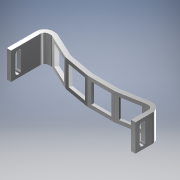
# Autodesk Inventor part: key_holder_metal
Saved by Autodesk Inventor 2018 (Build 220112000, 112)
## iProperties
Created: 2018-04-04
Part Number: key_holder_metal
Material: アルミニウム 6061
Document SubType Name: Sheet Metal
Designer: NaMACHAN
Density: 2.7 g/cm^3
Sheet Metal Rule: Default_mm
Appearance: アルミニウム - フラット
Mass: 6.46479 g
Surface Area: 40.6835 cm^2
Volume: 2.39437 cm^3
Author: NaMACHAN
Autodesk Inventor part; units mm, degrees
ref_plane "YZ Plane" through (0, 0, 0) normal (1, 0, 0) x (0, 1, 0)
ref_plane "XZ Plane" through (0, 0, 0) normal (0, 1, 0) x (-1, 0, 0)
ref_plane "XY Plane" through (0, 0, 0) normal (0, 0, 1) x (1, 0, 0)
sketch "スケッチ2" plane through (0, 0, 0) normal (0, 1, 0) x (-1, 0, 0)
  line L0 (-9.5, -9.5) -> (9.5, -9.5)
  line L1 (9.5, -9.5) -> (9.5, 9.5)
  line L2 (9.5, 9.5) -> (-9.5, 9.5)
  line L3 (-9.5, 9.5) -> (-9.5, -9.5)
  line L4 (-9.5, -9.5) -> (9.5, 9.5) construction
  line L5 (9.5, -9.5) -> (-9.5, 9.5) construction
  point P0 (0, 0)
  dimension "d4" = 19
  dimension "d5" = 19
  measures "d4" distance of L2.end L1.end
  measures "d5" distance of L1.end L0.end
extrude "プレート1" add sketch "スケッチ2" along normal blind 3
sketch "スケッチ3" plane through (8.9791, 2.9544, -9.5) normal (0.1736482, -0.9848078, 0) x (0.9848078, 0.1736482, 0)
  line L0 (0, 19) -> (0, 0)
  line L1 (0, 0) -> (19, 0)
  line L2 (19, 0) -> (19, 19)
  line L3 (19, 19) -> (0, 19)
  constraints: 6 end point, 1 horizontal, 1 perpendicular, 1 vertical
edge flange "フランジ1" height 19 angle 10 thickness 3 bend radius 3 thickness toward (0.1736482, -0.9848078, 0) relief straight relief width 3 relief depth 1.5 edges at (9.5, 3, 0) wall of the first edge with corners at (8.9791, 2.9544, 9.5) (8.9791, 2.9544, -9.5) (27.6904, 6.2537, -9.5) (27.6904, 6.2537, 9.5)
bend "曲げ1"
corner "コーナー1"
sketch "スケッチ4" plane through (-8.9791, 2.9544, 9.5) normal (-0.1736482, -0.9848078, 0) x (0.9848078, -0.1736482, 0)
  line L0 (0, -19) -> (0, 0)
  line L1 (0, 0) -> (-19, 0)
  line L2 (-19, 0) -> (-19, -19)
  line L3 (-19, -19) -> (0, -19)
  constraints: 6 end point, 1 horizontal, 1 perpendicular, 1 vertical
edge flange "フランジ2" height 19 angle 10 thickness 3 bend radius 3 thickness toward (-0.1736482, -0.9848078, 0) relief straight relief width 3 relief depth 1.5 edges at (-9.5, 3, 0) wall of the first edge with corners at (-8.9791, 2.9544, -9.5) (-8.9791, 2.9544, 9.5) (-27.6904, 6.2537, 9.5) (-27.6904, 6.2537, -9.5)
bend "曲げ2"
corner "コーナー2"
sketch "スケッチ5" plane through (-26.9435, 6.0182, 9.5) normal (-0.4226183, -0.9063078, 0) x (0.9063078, -0.4226183, 0)
  line L0 (0, -19) -> (0, 0)
  line L1 (0, 0) -> (-19.395, 0)
  line L2 (-19.395, 0) -> (-19.395, -19)
  line L3 (-19.395, -19) -> (0, -19)
  constraints: 6 end point, 1 horizontal, 1 perpendicular, 1 vertical
edge flange "フランジ3" height 19 angle 15 thickness 3 bend radius 3 thickness toward (-0.4226183, -0.9063078, 0) relief straight relief width 3 relief depth 1.5 edges at (-27.6904, 6.2537, 0) wall of the first edge with corners at (-26.9435, 6.0182, -9.5) (-26.9435, 6.0182, 9.5) (-44.5213, 14.2149, 9.5) (-44.5213, 14.2149, -9.5)
bend "曲げ3"
corner "コーナー3"
sketch "スケッチ11" plane through (9.496, 3.0456, 9.5) normal (-0.1736482, 0.9848078, 0) x (0.9848078, 0.1736482, 0)
  line L0 (0.9751, 17.5) -> (16.9751, 17.5)
  line L1 (16.9751, 17.5) -> (16.9751, 1.5)
  line L2 (16.9751, 1.5) -> (0.9751, 1.5)
  line L3 (0.9751, 1.5) -> (0.9751, 17.5)
  line L4 (0.9751, 17.5) -> (16.9751, 1.5) construction
  line L5 (16.9751, 17.5) -> (0.9751, 1.5) construction
  line L6 (18.4751, 0) -> (0, 0) projected
  line L7 (0, 19) -> (0, 0) projected
  point P0 (-9.8806, 9.5)
  point P1 (8.9751, 9.5)
  point P2 (8.9751, 9.5)
  point P3 (20.4467, 9.5)
  point P4 (8.9751, 9.5)
  point P5 (8.9751, 0)
  point P6 (17.9501, 0)
  point P7 (0, 9.5)
  dimension "d87" = 16
  dimension "d88" = 16
  constraints: 12 end point, 5 midpoint, 2 horizontal alignment, 2 parallel, 1 horizontal, 1 perpendicular, 1 point on line, 1 vertical alignment
  measures "d87" distance of L1.end L2.end
  measures "d88" distance of L0.end L1.end
extrude "押し出し2" cut sketch "スケッチ11" against normal blind 1.5
sketch "スケッチ12" plane through (0, 3, 0) normal (0, 1, 0) x (1, 0, 0)
  line L0 (-8, 8) -> (8, 8)
  line L1 (8, 8) -> (8, -8)
  line L2 (8, -8) -> (-8, -8)
  line L3 (-8, -8) -> (-8, 8)
  line L4 (-8, 8) -> (8, -8) construction
  line L5 (8, 8) -> (-8, -8) construction
  point P0 (0, 0)
  dimension "d91" = 16
  dimension "d92" = 16
  constraints: 12 end point, 2 midpoint, 2 parallel, 1 horizontal, 1 perpendicular
  measures "d91" distance of L1.end L2.end
  measures "d92" distance of L0.end L1.end
extrude "押し出し3" cut sketch "スケッチ12" against normal blind 1.5
sketch "スケッチ13" plane through (-9.496, 3.0456, 9.5) normal (0.1736482, 0.9848078, 0) x (0.9848078, -0.1736482, 0)
  line L0 (-0.8426, 17.5) -> (-16.8426, 17.5)
  line L1 (-16.8426, 17.5) -> (-16.8426, 1.5)
  line L2 (-16.8426, 1.5) -> (-0.8426, 1.5)
  line L3 (-0.8426, 1.5) -> (-0.8426, 17.5)
  line L4 (-0.8426, 17.5) -> (-16.8426, 1.5) construction
  line L5 (-16.8426, 17.5) -> (-0.8426, 1.5) construction
  line L6 (-17.6852, 19) -> (0, 19) projected
  line L7 (0.5209, 19) -> (0.5209, 0) projected
  point P0 (9.8806, 9.5)
  point P1 (-8.8426, 9.5)
  point P2 (-8.8426, 9.5)
  point P3 (-0.8426, 9.5)
  point P4 (-8.8426, 9.5)
  point P5 (-8.8426, 19)
  point P6 (0.5209, 9.5)
  dimension "d95" = 16
  dimension "d96" = 16
  constraints: 12 end point, 7 midpoint, 2 horizontal alignment, 2 parallel, 1 horizontal, 1 perpendicular, 1 vertical alignment
  measures "d95" distance of L2.end L1.end
  measures "d96" distance of L1.end L0.end
extrude "押し出し4" cut sketch "スケッチ13" against normal blind 1.5
sketch "スケッチ14" plane through (-27.6594, 6.3521, 9.5) normal (0.4226183, 0.9063078, 0) x (0.9063078, -0.4226183, 0)
  line L0 (-0.6374, 17.5) -> (-16.6374, 17.5)
  line L1 (-16.6374, 17.5) -> (-16.6374, 1.5)
  line L2 (-16.6374, 1.5) -> (-0.6374, 1.5)
  line L3 (-0.6374, 1.5) -> (-0.6374, 17.5)
  line L4 (-0.6374, 17.5) -> (-16.6374, 1.5) construction
  line L5 (-16.6374, 17.5) -> (-0.6374, 1.5) construction
  line L6 (-18.605, 19) -> (0, 19) projected
  line L7 (0, 0) -> (0, 19) projected
  point P0 (27.7524, 9.5)
  point P1 (-8.6374, 9.5)
  point P2 (-8.6374, 9.5)
  point P3 (-8.6374, 19)
  point P4 (-17.2749, 19)
  point P5 (-8.6374, 9.5)
  point P6 (0, 9.5)
  dimension "d99" = 16
  dimension "d100" = 16
  constraints: 12 end point, 5 midpoint, 2 parallel, 1 horizontal, 1 horizontal alignment, 1 perpendicular, 1 point on line, 1 vertical alignment
  measures "d99" distance of L2.end L1.end
  measures "d100" distance of L1.end L0.end
extrude "押し出し5" cut sketch "スケッチ14" against normal blind 1.5
sketch "スケッチ18" plane through (28.7323, 3.3449, -9.5) normal (0, 1, 0) x (1, 0, 0)
  line L0 (0, 19) -> (0, 0)
  line L1 (0, 0) -> (6.8755, 0)
  line L2 (6.8755, 0) -> (6.8755, 19)
  line L3 (6.8755, 19) -> (0, 19)
  constraints: 6 end point, 1 horizontal, 1 perpendicular, 1 vertical
edge flange "フランジ9" height 7.138 angle -10 thickness 3 bend radius 3 thickness toward (0, 1, 0) relief straight relief width 3 relief depth 1.5 edges at (27.6904, 6.2537, 0) wall of the first edge with corners at (28.7323, 3.3449, 9.5) (28.7323, 3.3449, -9.5) (35.6078, 3.3449, -9.5) (35.6078, 3.3449, 9.5)
bend "曲げ9"
corner "コーナー9"
sketch "スケッチ19" plane through (-47.057, 11.7771, 9.5) normal (0, 1, 0) x (1, 0, 0)
  line L0 (0, -19) -> (0, 0)
  line L1 (0, 0) -> (-7.3349, 0)
  line L2 (-7.3349, 0) -> (-7.3349, -19)
  line L3 (-7.3349, -19) -> (0, -19)
  constraints: 6 end point, 1 horizontal, 1 perpendicular, 1 vertical
edge flange "フランジ10" height 8 angle -25 thickness 3 bend radius 3 thickness toward (0, 1, 0) relief straight relief width 3 relief depth 1.5 edges at (-44.5213, 14.2149, 0) wall of the first edge with corners at (-47.057, 11.7771, -9.5) (-47.057, 11.7771, 9.5) (-54.3919, 11.7771, 9.5) (-54.3919, 11.7771, -9.5)
bend "曲げ10"
corner "コーナー10"
sketch "スケッチ20" plane through (32.6078, 6.3449, -9.5) normal (1, 0, 0) x (0, -1, 0)
  line L0 (0, 19) -> (0, 0)
  line L1 (0, 0) -> (18, 0)
  line L2 (18, 0) -> (18, 19)
  line L3 (18, 19) -> (0, 19)
  constraints: 6 end point, 1 horizontal, 1 perpendicular, 1 vertical
edge flange "フランジ11" height 15 angle -90 thickness 3 bend radius 3 thickness toward (1, 0, 0) relief straight relief width 3 relief depth 1.5 edges at (35.6078, 6.3449, 0) wall of the first edge with corners at (32.6078, 6.3449, 9.5) (32.6078, 6.3449, -9.5) (32.6078, -11.6551, -9.5) (32.6078, -11.6551, 9.5)
bend "曲げ11"
corner "コーナー11"
sketch "スケッチ21" plane through (-51.3919, 14.7771, 9.5) normal (-1, 0, 0) x (0, 1, 0)
  line L0 (0, -19) -> (0, 0)
  line L1 (0, 0) -> (-26.432, 0)
  line L2 (-26.432, 0) -> (-26.432, -19)
  line L3 (-26.432, -19) -> (0, -19)
  constraints: 6 end point, 1 horizontal, 1 perpendicular, 1 vertical
edge flange "フランジ12" height 23.432 angle -90 thickness 3 bend radius 3 thickness toward (-1, 0, 0) relief straight relief width 3 relief depth 1.5 edges at (-54.3919, 14.7771, 0) wall of the first edge with corners at (-51.3919, 14.7771, -9.5) (-51.3919, 14.7771, 9.5) (-51.3919, -11.6549, 9.5) (-51.3919, -11.6549, -9.5)
bend "曲げ12"
corner "コーナー12"
sketch "スケッチ22" plane through (35.6078, -11.6551, 9.5) normal (1, 0, 0) x (0, 0, -1)
  line L0 (4, 7) -> (15, 7)
  arc A0 (15, 3) -> (15, 7) centre (15, 5) ccw
  line L1 (15, 3) -> (4, 3)
  arc A1 (4, 7) -> (4, 3) centre (4, 5) ccw
  line L2 (0, 12) -> (0, 0) projected
  line L3 (19, 12) -> (19, 0) projected
  line L4 (0, 0) -> (19, 0) projected
  dimension "d194" = 2
  dimension "d195" = 4
  dimension "d196" = 4
  dimension "d197" = 5
  constraints: 4 end point, 4 point on circle, 4 tangent, 2 centre point, 1 horizontal, 1 parallel
  measures "d194" radius of A1
  measures "d195" distance from line of L2 A1.centre
  measures "d196" distance from line of L3 A0.centre
  measures "d197" distance from line of L4 A0.centre
extrude "押し出し8" cut sketch "スケッチ22" against normal blind 100
sketch "スケッチ23" plane through (9.7565, 1.5684, 9.5) normal (-0.1736482, 0.9848078, 0) x (0.9848078, 0.1736482, 0)
  line L0 (1.9751, 2.5) -> (15.9751, 2.5)
  line L1 (15.9751, 2.5) -> (15.9751, 16.5)
  line L2 (15.9751, 16.5) -> (1.9751, 16.5)
  line L3 (1.9751, 16.5) -> (1.9751, 2.5)
  line L4 (1.9751, 2.5) -> (15.9751, 16.5) construction
  line L5 (15.9751, 2.5) -> (1.9751, 16.5) construction
  line L6 (16.9751, 17.5) -> (16.9751, 1.5) projected
  line L7 (16.9751, 1.5) -> (0.9751, 1.5) projected
  point P0 (-9.8806, 9.5)
  point P1 (8.9751, 9.5)
  point P2 (8.9751, 9.5)
  point P3 (16.9751, 9.5)
  point P4 (8.9751, 9.5)
  point P5 (8.9751, 2.5)
  point P6 (8.9751, 1.5)
  dimension "d178" = 14
  dimension "d179" = 14
  constraints: 12 end point, 7 midpoint, 2 parallel, 2 vertical alignment, 1 horizontal, 1 horizontal alignment, 1 perpendicular
  measures "d178" distance of L2.end L1.end
  measures "d179" distance of L1.end L0.end
extrude "押し出し9" cut sketch "スケッチ23" against normal blind 1.5
sketch "スケッチ24" plane through (0, 1.5, 0) normal (0, 1, 0) x (1, 0, 0)
  line L0 (-7, -7) -> (7, -7)
  line L1 (7, -7) -> (7, 7)
  line L2 (7, 7) -> (-7, 7)
  line L3 (-7, 7) -> (-7, -7)
  line L4 (-7, -7) -> (7, 7) construction
  line L5 (7, -7) -> (-7, 7) construction
  point P0 (0, 0)
  dimension "d182" = 14
  dimension "d183" = 14
  constraints: 12 end point, 2 midpoint, 2 parallel, 1 horizontal, 1 perpendicular
  measures "d182" distance of L2.end L1.end
  measures "d183" distance of L1.end L0.end
extrude "押し出し10" cut sketch "スケッチ24" against normal blind 1.5
sketch "スケッチ25" plane through (-9.7565, 1.5684, 9.5) normal (0.1736482, 0.9848078, 0) x (0.9848078, -0.1736482, 0)
  line L0 (-15.8426, 2.5) -> (-1.8426, 2.5)
  line L1 (-1.8426, 2.5) -> (-1.8426, 16.5)
  line L2 (-1.8426, 16.5) -> (-15.8426, 16.5)
  line L3 (-15.8426, 16.5) -> (-15.8426, 2.5)
  line L4 (-15.8426, 2.5) -> (-1.8426, 16.5) construction
  line L5 (-1.8426, 2.5) -> (-15.8426, 16.5) construction
  line L6 (-0.8426, 1.5) -> (-16.8426, 1.5) projected
  line L7 (-0.8426, 17.5) -> (-0.8426, 1.5) projected
  point P0 (9.8806, 9.5)
  point P1 (-8.8426, 9.5)
  point P2 (-8.8426, 9.5)
  point P3 (-8.8426, 1.5)
  point P4 (-8.8426, 9.5)
  point P5 (-0.8426, 9.5)
  dimension "d186" = 14
  dimension "d187" = 14
  constraints: 12 end point, 6 midpoint, 2 parallel, 1 horizontal, 1 horizontal alignment, 1 perpendicular, 1 vertical alignment
  measures "d186" distance of L2.end L1.end
  measures "d187" distance of L1.end L0.end
extrude "押し出し11" cut sketch "スケッチ25" against normal blind 1.5
sketch "スケッチ26" plane through (-28.2933, 4.9926, 9.5) normal (0.4226183, 0.9063078, 0) x (0.9063078, -0.4226183, 0)
  line L0 (-15.6374, 2.5) -> (-1.6374, 2.5)
  line L1 (-1.6374, 2.5) -> (-1.6374, 16.5)
  line L2 (-1.6374, 16.5) -> (-15.6374, 16.5)
  line L3 (-15.6374, 16.5) -> (-15.6374, 2.5)
  line L4 (-15.6374, 2.5) -> (-1.6374, 16.5) construction
  line L5 (-1.6374, 2.5) -> (-15.6374, 16.5) construction
  line L6 (-0.6374, 1.5) -> (-16.6374, 1.5) projected
  line L7 (-0.6374, 17.5) -> (-0.6374, 1.5) projected
  point P0 (27.7524, 9.5)
  point P1 (-8.6374, 9.5)
  point P2 (-8.6374, 9.5)
  point P3 (-8.6374, 1.5)
  point P4 (-8.6374, 9.5)
  point P5 (-0.6374, 9.5)
  dimension "d190" = 14
  dimension "d191" = 14
  constraints: 12 end point, 6 midpoint, 2 parallel, 1 horizontal, 1 horizontal alignment, 1 perpendicular, 1 vertical alignment
  measures "d190" distance of L2.end L1.end
  measures "d191" distance of L1.end L0.end
extrude "押し出し12" cut sketch "スケッチ26" against normal blind 1.5
equation "\"d6\" = Thickness"
equation "\"d7\" = BendReliefWidth"
equation "\"d8\" = BendReliefDepth"
equation "\"d9\" = MinimumRemnant"
equation "\"d10\" = TransitionRadius"
equation "\"d13\" = BendRadius"
equation "\"d14\" = CornerReliefSize"
equation "\"d15\" = GapSize"
equation "\"d16\" = JacobiRadiusSize"
equation "\"d17\" = BendReliefWidth"
equation "\"d18\" = BendReliefDepth"
equation "\"d19\" = MinimumRemnant"
equation "\"d20\" = TransitionRadius"
equation "\"d23\" = BendRadius"
equation "\"d24\" = CornerReliefSize"
equation "\"d25\" = GapSize"
equation "\"d26\" = JacobiRadiusSize"
equation "\"d27\" = BendReliefWidth"
equation "\"d28\" = BendReliefDepth"
equation "\"d29\" = MinimumRemnant"
equation "\"d30\" = TransitionRadius"
equation "\"d33\" = BendRadius"
equation "\"d34\" = CornerReliefSize"
equation "\"d35\" = GapSize"
equation "\"d36\" = JacobiRadiusSize"
equation "\"d133\" = BendReliefWidth"
equation "\"d134\" = BendReliefDepth"
equation "\"d135\" = MinimumRemnant"
equation "\"d136\" = TransitionRadius"
equation "\"d139\" = BendRadius"
equation "\"d140\" = CornerReliefSize"
equation "\"d141\" = GapSize"
equation "\"d142\" = JacobiRadiusSize"
equation "\"d143\" = BendReliefWidth"
equation "\"d144\" = BendReliefDepth"
equation "\"d145\" = MinimumRemnant"
equation "\"d146\" = TransitionRadius"
equation "\"d149\" = BendRadius"
equation "\"d150\" = CornerReliefSize"
equation "\"d151\" = GapSize"
equation "\"d152\" = JacobiRadiusSize"
equation "\"d153\" = BendReliefWidth"
equation "\"d154\" = BendReliefDepth"
equation "\"d155\" = MinimumRemnant"
equation "\"d156\" = TransitionRadius"
equation "\"d159\" = BendRadius"
equation "\"d160\" = CornerReliefSize"
equation "\"d161\" = GapSize"
equation "\"d162\" = JacobiRadiusSize"
equation "\"d163\" = BendReliefWidth"
equation "\"d164\" = BendReliefDepth"
equation "\"d165\" = MinimumRemnant"
equation "\"d166\" = TransitionRadius"
equation "\"d169\" = BendRadius"
equation "\"d170\" = CornerReliefSize"
equation "\"d171\" = GapSize"
equation "\"d172\" = JacobiRadiusSize"
equation "\"BendRadius\" = Thickness"
equation "\"BendReliefWidth\" = Thickness"
equation "\"BendReliefDepth\" = 0.5 * Thickness"
equation "\"CornerReliefSize\" = 4 * Thickness"
equation "\"MinimumRemnant\" = 2 * Thickness"
equation "\"TransitionRadius\" = BendRadius"
equation "\"JacobiRadiusSize\" = BendRadius"
equation "\"GapSize\" = Thickness"
equation "\"Thickness\" = 3"
